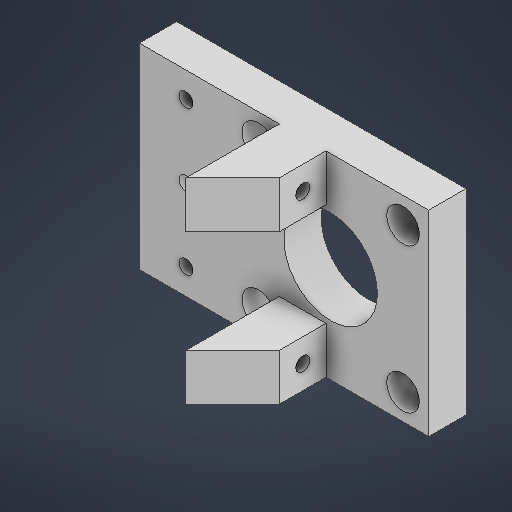
# Autodesk Inventor part: end motor holder
Saved by Autodesk Inventor 2025.1 (Build 291241000, 241)
## iProperties
Created: 2025-02-02
Part Number: end motor holder
Material: Generic
Document SubType Name: Modeling
Designer: jerem
Density: 1 g/cm^3
Appearance: Default
Author: jerem
Autodesk Inventor part; units mm, degrees
ref_plane "YZ Plane" through (0, 0, 0) normal (1, 0, 0) x (0, 1, 0)
ref_plane "XZ Plane" through (0, 0, 0) normal (0, 1, 0) x (-1, 0, 0)
ref_plane "XY Plane" through (0, 0, 0) normal (0, 0, 1) x (1, 0, 0)
sketch "Sketch1" plane through (0, 0, 0) normal (0, 0, 1) x (1, 0, 0)
  line L0 (21, -21) -> (-21, -21)
  line L1 (-21, -21) -> (-21, 21)
  line L2 (-21, 21) -> (21, 21)
  line L3 (21, 21) -> (21, -21)
  line L4 (21, -21) -> (-21, 21) construction
  line L5 (-21, -21) -> (21, 21) construction
  circle A0 centre (-15.5, 15.5) radius 1.5
  circle A1 centre (15.5, 15.5) radius 1.5
  circle A2 centre (15.5, -15.5) radius 1.5
  circle A3 centre (-15.5, -15.5) radius 1.5
  line L6 (-15.5, 15.5) -> (-15.5, -15.5) construction
  line L7 (-15.5, 15.5) -> (15.5, 15.5) construction
  line L8 (15.5, 15.5) -> (15.5, -15.5) construction
  circle A4 centre (-15.5, 15.5) radius 4.5
  circle A5 centre (15.5, 15.5) radius 4.5
  circle A6 centre (15.5, -15.5) radius 4.5
  circle A7 centre (-15.5, -15.5) radius 4.5
  circle A8 centre (0, 0) radius 10
  dimension "d0" = 42
  dimension "d1" = 42
  dimension "d2" = 31
  dimension "d3" = 3
  dimension "d4" = 3
  dimension "d7" = 20
  constraints: 18 end point, 9 centre point, 6 equal radius, 4 point on line, 3 parallel, 2 midpoint, 2 perpendicular, 1 coincident, 1 horizontal, 1 vertical
  measures "d0" distance of L1.end L2.end
  measures "d1" distance of L0.end L1.end
  measures "d2" distance of L6.start L7.end
  measures "d3" diameter of A0
  measures "d4" radial gap between concentric circles of A4 A0
  measures "d7" diameter of A8
extrude "Extrusion1" add sketch "Sketch1" along normal blind 8 contours L0 L1 L2 L3 | A4 | A5 | A6 | A7
sketch "Sketch2" plane through (0, 0, 8) normal (0, 0, 1) x (1, 0, 0)
  line L0 (21, 21) -> (-21, 21) projected
  line L1 (-21, 21) -> (-21, -21) projected
  line L2 (-21, -21) -> (21, -21) projected
  line L3 (21, -21) -> (21, 21) projected
  circle A0 centre (-15.5, 15.5) radius 1.5 projected
  circle A1 centre (15.5, 15.5) radius 1.5 projected
  circle A2 centre (15.5, -15.5) radius 1.5 projected
  circle A3 centre (0, 0) radius 10 projected
  circle A4 centre (-15.5, -15.5) radius 1.5 projected
  circle A5 centre (-15.5, 15.5) radius 3.5
  circle A6 centre (15.5, 15.5) radius 3.5
  circle A7 centre (15.5, -15.5) radius 3.5
  circle A8 centre (-15.5, -15.5) radius 3.5
  dimension "d10" = 7
  constraints: 4 centre point, 4 coincident, 3 equal radius
  measures "d10" diameter of A5
extrude "Extrusion3" cut sketch "Sketch2" against normal blind 5 contours A5 | A6 | A7 | A8
sketch "Sketch3" plane through (0, 0, 8) normal (0, 0, 1) x (1, 0, 0)
  circle A0 centre (15.5, -15.5) radius 3.5 projected
  circle A1 centre (15.5, 15.5) radius 3.5 projected
  circle A2 centre (-15.5, -15.5) radius 3.5 projected
  circle A3 centre (-15.5, 15.5) radius 3.5 projected
  line L0 (21, 21) -> (-21, 21) projected
  line L1 (-21, 21) -> (-21, -21) projected
  line L2 (-21, -21) -> (21, -21) projected
  line L3 (21, -21) -> (21, 21) projected
  circle A4 centre (0, 0) radius 10 projected
  line L4 (-11, 21) -> (-11, -21)
  line L5 (-11, 11) -> (-1, 11)
  line L6 (-1, 11) -> (-1, 21)
  line L7 (-11, -11) -> (-1, -11)
  line L8 (-1, -11) -> (-1, -21)
  dimension "d13" = 10
  dimension "d14" = 10
  dimension "d15" = 10
  constraints: 10 end point, 6 point on line, 3 perpendicular, 2 equal length, 2 horizontal
  measures "d13" distance between parallel lines of L1 L4
  measures "d14" distance of L5.end L6.end
  measures "d15" distance of L5.start L5.end
extrude "Extrusion4" add sketch "Sketch3" along normal blind 10 contours L6 L5 L4 L0 | L2 L4 L7 L8
sketch "Sketch4" plane through (0, 0, 0) normal (0, 0, -1) x (-1, 0, 0)
  line L0 (21, 21) -> (21, -21) projected
  line L1 (21, 21) -> (41, 21)
  line L2 (41, 21) -> (41, -21)
  line L3 (41, -21) -> (21, -21)
  circle A0 centre (31, 15.5) radius 1.5
  circle A1 centre (31, -15.5) radius 1.5
  line L4 (31, 15.5) -> (31, -15.5) construction
  line L5 (31, 0) -> (21, 0) construction
  circle A2 centre (31, 0) radius 1.5
  point P0 (0, 0)
  dimension "d18" = 31
  dimension "d19" = 10
  dimension "d20" = 10
  dimension "d21" = 3
  constraints: 10 end point, 3 centre point, 3 perpendicular, 2 equal radius, 2 midpoint, 1 coincident, 1 horizontal, 1 vertical
  measures "d18" distance of L4.start L4.end
  measures "d19" distance of L5.start L5.end
  measures "d20" distance between parallel lines of L4 L2
  measures "d21" diameter of A0
extrude "Extrusion5" add sketch "Sketch4" against normal up to surface (8 mm away)
sketch "Sketch5" plane through (-11, 11, 8) normal (-1, 0, 0) x (0, 0, 1)
  line L0 (0, 0) -> (0, 10) projected
  line L1 (0, 0) -> (10, 0) projected
  line L2 (10, 10) -> (10, 0) projected
  line L3 (0, 10) -> (10, 10) projected
  line L4 (0, -32) -> (0, -22) projected
  line L5 (0, -32) -> (10, -32) projected
  line L6 (10, -22) -> (10, -32) projected
  line L7 (0, -22) -> (10, -22) projected
  line L8 (10, 10) -> (0, 0) construction
  line L9 (10, 0) -> (0, 10) construction
  line L10 (10, -32) -> (0, -22) construction
  line L11 (10, -22) -> (0, -32) construction
  circle A0 centre (5, 5) radius 1.5
  circle A1 centre (5, -27) radius 1.5
  point P0 (-8, -11)
  dimension "d24" = 3
  dimension "d25" = 3
  constraints: 8 end point, 2 centre point, 2 midpoint, 2 perpendicular, 1 parallel
  measures "d24" diameter of A0
  measures "d25" diameter of A1
extrude "Extrusion6" cut sketch "Sketch5" against normal through all contours A0 | A1
draft "FaceDraft1" angle 45 pull direction (1, 0, 0) faces at (-7.6667, -14.3333, 18) (-7.6667, 17.6667, 18) fixed edges at (-1, -16, 18) (-1, 16, 18)
body "Solid1"
